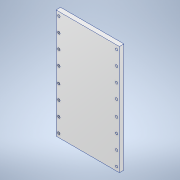
# Autodesk Inventor part: actuatorMount
Saved by Autodesk Inventor 2021 (Build 250183000, 183)
## iProperties
Created: 2021-03-21
Part Number: actuatorMount
Material: Aluminum 6061
Document SubType Name: Modeling
Designer: Work
Mass: 1829.05 g
Surface Area: 1231.3 cm^2
Volume: 677.425 cm^3
Density: 2.7 g/cm^3
Appearance: Aluminum - Flat
Author: Work
Autodesk Inventor part; units mm, degrees
ref_plane "YZ Plane" through (0, 0, 0) normal (1, 0, 0) x (0, 1, 0)
ref_plane "XZ Plane" through (0, 0, 0) normal (0, 1, 0) x (-1, 0, 0)
ref_plane "XY Plane" through (0, 0, 0) normal (0, 0, 1) x (1, 0, 0)
sketch "Sketch1" plane through (0, 0, 0) normal (0, 0, 1) x (1, 0, 0)
  line L0 (0, 0) -> (176.8, 0)
  line L1 (176.8, 0) -> (176.8, 304.8)
  line L2 (176.8, 304.8) -> (0, 304.8)
  line L3 (0, 304.8) -> (0, 0)
  dimension "d1" = 176.8
  dimension "d2" = 304.8
  constraints: 8 end point, 2 parallel, 1 horizontal, 1 perpendicular
  measures "d1" distance of L1.end L2.end
  measures "d2" distance of L0.end L1.end
extrude "Extrusion1" add sketch "Sketch1" along normal blind 12.7
sketch "Sketch2" plane through (0, 0, 12.7) normal (0, 0, 1) x (1, 0, 0)
  line L0 (0, 0) -> (176.8, 0) projected
  line L1 (0, 304.8) -> (0, 0) projected
  point P0 (8, 11)
  point P1 (8, 51)
  point P2 (8, 91)
  point P3 (8, 131)
  dimension "d5" = 40
  dimension "d6" = 40
  dimension "d7" = 40
  dimension "d8" = 11
  dimension "d9" = 8
  measures "d5" distance of point (8, 51) point (8, 11)
  measures "d6" distance of point (8, 51) point (8, 91)
  measures "d7" distance of point (8, 91) point (8, 131)
  measures "d8" distance from line of L0 point (8, 11)
  measures "d9" distance from line of L1 point (8, 11)
hole "Hole1" at (8, 11, 12.7) at (8, 51, 12.7) at (8, 91, 12.7) at (8, 131, 12.7) direction (0, 0, -1) diameter 6.604 end through all clearance for "Socket Head Cap Screw" size "M6" standard "Ansi Metric M Profile"
pattern_linear "Rectangular Pattern1" count 2 spacing 162.8 along (0, 1, 0) count 2 spacing 161 along (1, 0, 0) of "Hole1"
body "Solid1"
